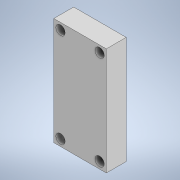
# Autodesk Inventor part: Ch7(5) Part 9 Cover Plate
Saved by Autodesk Inventor 2020 (Build 240168000, 168)
## iProperties
Created: 2021-03-04
Part Number: Ch7(5) Part 9 Cover Plate
Material: Generic
Document SubType Name: Modeling
Designer: adriggs
Density: 1 g/cm^3
Appearance: Default
Author: adriggs
Autodesk Inventor part; units mm, degrees
ref_plane "YZ Plane" through (0, 0, 0) normal (1, 0, 0) x (0, 1, 0)
ref_plane "XZ Plane" through (0, 0, 0) normal (0, 1, 0) x (-1, 0, 0)
ref_plane "XY Plane" through (0, 0, 0) normal (0, 0, 1) x (1, 0, 0)
sketch "Sketch1" plane through (0, 0, 0) normal (0, 0, 1) x (1, 0, 0)
  line L0 (-12.4142, 25.4) -> (12.4142, 25.4)
  line L1 (12.4142, 25.4) -> (12.4142, -25.4)
  line L2 (12.4142, -25.4) -> (-12.4142, -25.4)
  line L3 (-12.4142, -25.4) -> (-12.4142, 25.4)
  circle A0 centre (-9.2393, 22.225) radius 2.1844
  circle A1 centre (-9.2393, -22.225) radius 2.1844
  circle A2 centre (9.2393, -22.225) radius 2.1844
  circle A3 centre (9.2393, 22.225) radius 2.1844
  point P0 (0, 0)
  point P1 (-12.4143, 0)
  point P2 (0, 25.4)
  dimension "d0" = 24.8285
  dimension "d1" = 50.8
  dimension "d2" = 4.3688
  dimension "d3" = 47.625
  dimension "d4" = 3.175
  dimension "d5" = 4.3688
  dimension "d6" = 4.3688
  dimension "d7" = 4.3688
  dimension "d8" = 3.175
  dimension "d9" = 3.175
  constraints: 8 end point, 4 centre point, 3 horizontal alignment, 3 vertical alignment, 2 midpoint, 2 parallel, 1 horizontal, 1 perpendicular
  measures "d0" distance of L1.end L2.end
  measures "d1" distance of L0.end L1.end
  measures "d2" diameter of A0
  measures "d3" vertical distance of A0.centre L2.end
  measures "d4" distance from line of L3 A0.centre
  measures "d5" diameter of A1
  measures "d6" diameter of A2
  measures "d7" diameter of A3
  measures "d8" distance from line of L1 A3.centre
  measures "d9" horizontal distance of L1.end A2.centre
extrude "Extrusion1" add sketch "Sketch1" against normal blind 9.398
body "Solid1"
